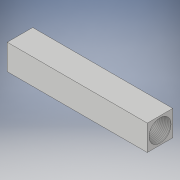
# Autodesk Inventor part: 2nd arm
Saved by Autodesk Inventor 2017 (Build 210142000, 142)
## iProperties
Created: 2020-02-04
Part Number: 2nd arm
Material: Generic
Document SubType Name: Modeling
Designer: S346852600
Density: 1 g/cm^3
Appearance: Default
Author: S346852600
Autodesk Inventor part; units mm, degrees
ref_plane "YZ Plane" through (0, 0, 0) normal (1, 0, 0) x (0, 1, 0)
ref_plane "XZ Plane" through (0, 0, 0) normal (0, 1, 0) x (-1, 0, 0)
ref_plane "XY Plane" through (0, 0, 0) normal (0, 0, 1) x (1, 0, 0)
sketch "Sketch1" plane through (0, 0, 0) normal (1, 0, 0) x (0, 1, 0)
  line L0 (1.2978, 13.4356) -> (26.6978, 13.4356)
  line L1 (26.6978, 13.4356) -> (26.6978, -11.9644)
  line L2 (26.6978, -11.9644) -> (1.2978, -11.9644)
  line L3 (1.2978, -11.9644) -> (1.2978, 13.4356)
  line L4 (24.1578, -9.4244) -> (24.1578, 10.8956)
  line L5 (24.1578, 10.8956) -> (3.8378, 10.8956)
  line L6 (3.8378, 10.8956) -> (3.8378, -9.4244)
  line L7 (3.8378, -9.4244) -> (24.1578, -9.4244)
  point P0 (0, 0)
  dimension "d0" = 25.4
  dimension "d1" = 25.4
  dimension "d2" = 2.54
  constraints: 16 end point, 4 parallel, 2 perpendicular, 1 horizontal, 3 other
  measures "d0" distance of L1.end L2.end
  measures "d1" distance of L0.end L1.end
  measures "d2" distance between parallel lines of L1 L4
extrude "Extrusion1" add sketch "Sketch1" along normal blind 139.7
sketch "Sketch2" plane through (0, 3.8378, -9.4244) normal (0, 0, 1) x (1, 0, 0)
  line L0 (0, 0) -> (139.7, 0) projected
  line L1 (139.7, 0) -> (118.618, 0)
  line L2 (118.618, 0) -> (118.618, 20.32)
  line L3 (118.618, 20.32) -> (139.7, 20.32)
  line L4 (139.7, 20.32) -> (139.7, 0)
  point P0 (0, -3.8378)
  dimension "d5" = 21.082
  dimension "d6" = 20.32
  constraints: 8 end point, 2 parallel, 1 horizontal, 1 perpendicular
  measures "d5" distance of L2.end L3.end
  measures "d6" distance of L1.end L2.end
extrude "Extrusion2" add sketch "Sketch2" along normal blind 20.32
sketch "Sketch3" plane through (139.7, 0, 0) normal (1, 0, 0) x (0, 0, -1)
  line L0 (11.9644, 1.2978) -> (-13.4356, 1.2978) projected
  line L1 (-0.7356, 1.2978) -> (-0.7356, 13.9978)
  line L2 (-13.4356, 26.6978) -> (11.9644, 26.6978) projected
  circle A0 centre (-0.7356, 13.9978) radius 10.9855
  point P0 (0, 0)
  dimension "d9" = 12.7
  dimension "d10" = 21.971
  constraints: 2 end point, 1 centre point, 1 coincident, 1 midpoint, 1 perpendicular
  measures "d9" distance of L1.start L1.end
  measures "d10" diameter of A0
extrude "Extrusion3" cut sketch "Sketch3" against normal blind 21.082
thread "Thread1" size "M22x1.5" class "6H" standard "ANSI Metric M Profile" full length
body "Solid1"
